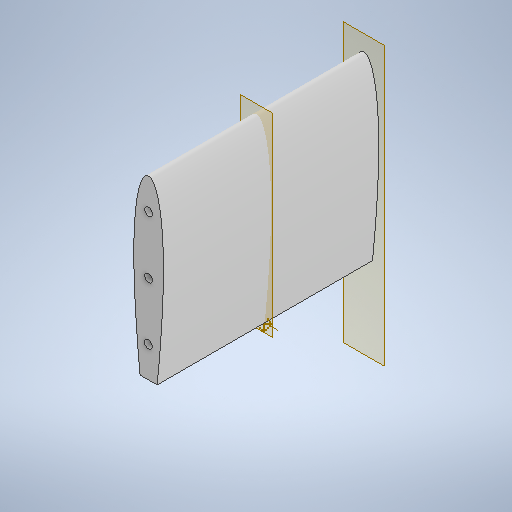
# Autodesk Inventor part: MiddleTailLeft
Saved by Autodesk Inventor 2025.2 (Build 292293000, 293)
## iProperties
Created: 2025-03-03
Part Number: MiddleTailLeft
Material: Generic
Document SubType Name: Modeling
Designer: georg
Density: 1 g/cm^3
Appearance: Default
Author: georg
Autodesk Inventor part; units mm, degrees
ref_plane "YZ Plane" through (0, 0, 0) normal (1, 0, 0) x (0, 1, 0)
ref_plane "XZ Plane" through (0, 0, 0) normal (0, 1, 0) x (-1, 0, 0)
ref_plane "XY Plane" through (0, 0, 0) normal (0, 0, 1) x (1, 0, 0)
ref_plane "Work Plane1" through (0, 0, 156.21) normal (0, 0, 1) x (1, 0, 0)
sketch "Sketch1" plane through (0, 0, 156.21) normal (0, 0, 1) x (1, 0, 0)
  line L0 (-0.0073, -145.66) -> (7.0407, -145.66)
  spline S0 degree 5 poles (7.0407, -145.66) (7.0573, -145.4958) (7.1327, -144.7531) (7.2665, -143.4248) (7.4579, -141.501) (7.705, -138.9697) (7.9903, -135.9869) (8.2715, -132.9695) (8.549, -129.922) (8.8215, -126.8457) (9.0881, -123.745) (9.3491, -120.6224) (9.6026, -117.4806) (9.8495, -114.3238) (10.0866, -111.1538) (10.3164, -107.9748) (10.5349, -104.7893) (10.7445, -101.6008) (10.942, -98.4123) (11.1277, -95.2267) (11.3009, -92.0477) (11.4615, -88.8777) (11.6069, -85.7208) (11.739, -82.5791) (11.8548, -79.4563) (11.9554, -76.3556) (12.039, -73.2792) (12.1057, -70.2316) (12.1549, -67.2141) (12.1854, -64.2311) (12.198, -61.2847) (12.1911, -58.378) (12.1652, -55.5142) (12.1197, -52.6956) (12.0539, -49.9253) (11.9681, -47.2063) (11.8622, -44.5404) (11.7355, -41.9312) (11.589, -39.3806) (11.4216, -36.8917) (11.2342, -34.4665) (11.0264, -32.1073) (10.7996, -29.817) (10.5524, -27.5973) (10.2861, -25.4503) (10.0015, -23.3788) (9.698, -21.3841) (9.3765, -19.469) (9.0379, -17.6343) (8.682, -15.8826) (8.3103, -14.2152) (7.9227, -12.634) (7.5202, -11.1404) (7.103, -9.7353) (6.6725, -8.4212) (6.2284, -7.198) (5.7722, -6.0677) (5.3036, -5.0307) (4.8237, -4.0882) (4.3332, -3.2402) (3.831, -2.4886) (3.3186, -1.832) (2.7948, -1.2726) (2.2592, -0.8103) (1.7116, -0.4465) (1.151, -0.1846) (0.5803, -0.0264) (0, 0.026) (-0.5803, -0.0264) (-1.151, -0.1846) (-1.7116, -0.4465) (-2.2592, -0.8103) (-2.7948, -1.2726) (-3.3186, -1.832) (-3.831, -2.4886) (-4.3332, -3.2402) (-4.8237, -4.0882) (-5.3036, -5.0307) (-5.7722, -6.0677) (-6.2284, -7.198) (-6.6725, -8.4212) (-7.103, -9.7353) (-7.5202, -11.1404) (-7.9227, -12.634) (-8.3103, -14.2152) (-8.682, -15.8826) (-9.0379, -17.6343) (-9.3765, -19.469) (-9.698, -21.3841) (-10.0015, -23.3788) (-10.2861, -25.4503) (-10.5524, -27.5973) (-10.7996, -29.817) (-11.0264, -32.1073) (-11.2342, -34.4665) (-11.4216, -36.8917) (-11.589, -39.3806) (-11.7355, -41.9312) (-11.8622, -44.5404) (-11.9681, -47.2063) (-12.0539, -49.9253) (-12.1197, -52.6956) (-12.1652, -55.5142) (-12.1911, -58.378) (-12.198, -61.2847) (-12.1854, -64.2311) (-12.1549, -67.2141) (-12.1057, -70.2316) (-12.039, -73.2792) (-11.9554, -76.3556) (-11.8548, -79.4563) (-11.739, -82.5791) (-11.6069, -85.7208) (-11.4615, -88.8777) (-11.3009, -92.0477) (-11.1277, -95.2267) (-10.942, -98.4123) (-10.7445, -101.6008) (-10.5349, -104.7893) (-10.3164, -107.9748) (-10.0866, -111.1538) (-9.8495, -114.3238) (-9.6026, -117.4806) (-9.3491, -120.6224) (-9.0881, -123.745) (-8.8215, -126.8457) (-8.549, -129.922) (-8.2715, -132.9695) (-7.9903, -135.9869) (-7.705, -138.9697) (-7.4579, -141.501) (-7.2665, -143.4248) (-7.1327, -144.7531) (-7.0573, -145.4958) (-7.0407, -145.66) knots 0.155732 0.155732 0.155732 0.155732 0.155732 0.155732 0.15748 0.163633 0.169829 0.176062 0.18233 0.188629 0.194957 0.201309 0.207683 0.214076 0.220484 0.226904 0.233333 0.239767 0.246204 0.25264 0.259072 0.265497 0.271912 0.278314 0.284699 0.291064 0.297407 0.303723 0.310011 0.316266 0.322485 0.328666 0.334804 0.340898 0.346943 0.352937 0.358876 0.364757 0.370576 0.376331 0.382017 0.387632 0.393172 0.398634 0.404014 0.409309 0.414515 0.419627 0.424644 0.42956 0.434371 0.439075 0.443667 0.448142 0.452498 0.456729 0.460831 0.464802 0.468638 0.472335 0.475892 0.479309 0.482586 0.485731 0.488751 0.491664 0.494492 0.497262 0.5 0.502738 0.505508 0.508336 0.511249 0.514269 0.517414 0.520691 0.524108 0.527665 0.531362 0.535198 0.539169 0.543271 0.547502 0.551858 0.556333 0.560925 0.565629 0.57044 0.575356 0.580373 0.585485 0.590691 0.595986 0.601366 0.606828 0.612368 0.617983 0.623669 0.629424 0.635243 0.641124 0.647063 0.653057 0.659102 0.665196 0.671334 0.677515 0.683734 0.689989 0.696277 0.702593 0.708936 0.715301 0.721686 0.728088 0.734503 0.740928 0.74736 0.753796 0.760233 0.766667 0.773096 0.779516 0.785924 0.792317 0.798691 0.805043 0.811371 0.81767 0.823938 0.830171 0.836367 0.84252 0.844268 0.844268 0.844268 0.844268 0.844268 0.844268
  line L1 (-7.0407, -145.66) -> (-0.0073, -145.66)
  point P0 (0, 0)
  point P1 (7.4123, -141.9502)
  point P2 (7.7005, -139.0014)
  point P3 (7.9858, -136.0158)
  point P4 (8.2674, -132.996)
  point P5 (8.545, -129.9456)
  point P6 (8.8177, -126.8669)
  point P7 (9.0847, -123.7634)
  point P8 (9.3456, -120.638)
  point P9 (9.5996, -117.4937)
  point P10 (9.8461, -114.3339)
  point P11 (10.084, -111.1614)
  point P12 (10.3132, -107.9795)
  point P13 (10.5325, -104.7913)
  point P14 (10.7416, -101.6)
  point P15 (10.9393, -98.4087)
  point P16 (11.125, -95.2205)
  point P17 (11.2983, -92.0386)
  point P18 (11.4584, -88.8661)
  point P19 (11.6043, -85.7063)
  point P20 (11.7358, -82.562)
  point P21 (11.8518, -79.4366)
  point P22 (11.952, -76.3331)
  point P23 (12.0355, -73.2544)
  point P24 (12.102, -70.204)
  point P25 (12.1508, -67.1842)
  point P26 (12.1812, -64.1986)
  point P27 (12.1932, -61.2498)
  point P28 (12.1861, -58.3408)
  point P29 (12.1597, -55.4746)
  point P30 (12.1136, -52.6538)
  point P31 (12.0473, -49.8813)
  point P32 (11.961, -47.1601)
  point P33 (11.8543, -44.4923)
  point P34 (11.7271, -41.8809)
  point P35 (11.5796, -39.3285)
  point P36 (11.4115, -36.8377)
  point P37 (11.2231, -34.4107)
  point P38 (11.0147, -32.0499)
  point P39 (10.7865, -29.758)
  point P40 (10.5384, -27.5369)
  point P41 (10.2709, -25.3886)
  point P42 (9.9848, -23.3158)
  point P43 (9.68, -21.3202)
  point P44 (9.3572, -19.404)
  point P45 (9.0168, -17.5687)
  point P46 (8.6594, -15.8163)
  point P47 (8.2857, -14.1486)
  point P48 (7.8961, -12.5673)
  point P49 (7.4914, -11.0738)
  point P50 (7.072, -9.6695)
  point P51 (6.6387, -8.3562)
  point P52 (6.1921, -7.1348)
  point P53 (5.7329, -6.0066)
  point P54 (5.2615, -4.9727)
  point P55 (4.7787, -4.0341)
  point P56 (4.2851, -3.1919)
  point P57 (3.7809, -2.4469)
  point P58 (3.267, -1.7995)
  point P59 (2.7438, -1.2509)
  point P60 (2.2116, -0.8012)
  point P61 (1.6709, -0.4509)
  point P62 (1.1219, -0.2006)
  point P63 (0.5647, -0.0502)
  point P64 (0, 0)
  point P65 (-0.5647, -0.0502)
  point P66 (-1.1219, -0.2006)
  point P67 (-1.6709, -0.4509)
  point P68 (-2.2116, -0.8012)
  point P69 (-2.7438, -1.2509)
  point P70 (-3.267, -1.7995)
  point P71 (-3.7809, -2.4469)
  point P72 (-4.2851, -3.1919)
  point P73 (-4.7787, -4.0341)
  point P74 (-5.2615, -4.9727)
  point P75 (-5.7329, -6.0066)
  point P76 (-6.1921, -7.1348)
  point P77 (-6.6387, -8.3562)
  point P78 (-7.072, -9.6695)
  point P79 (-7.4914, -11.0738)
  point P80 (-7.8961, -12.5673)
  point P81 (-8.2857, -14.1486)
  point P82 (-8.6594, -15.8163)
  point P83 (-9.0168, -17.5687)
  point P84 (-9.3572, -19.404)
  point P85 (-9.68, -21.3202)
  point P86 (-9.9848, -23.3158)
  point P87 (-10.2709, -25.3886)
  point P88 (-10.5384, -27.5369)
  point P89 (-10.7865, -29.758)
  point P90 (-11.0147, -32.0499)
  point P91 (-11.2231, -34.4107)
  point P92 (-11.4115, -36.8377)
  point P93 (-11.5796, -39.3285)
  point P94 (-11.7271, -41.8809)
  point P95 (-11.8543, -44.4923)
  point P96 (-11.961, -47.1601)
  point P97 (-12.0473, -49.8813)
  point P98 (-12.1136, -52.6538)
  point P99 (-12.1597, -55.4746)
  point P100 (-12.1861, -58.3408)
  point P101 (-12.1932, -61.2498)
  point P102 (-12.1812, -64.1986)
  point P103 (-12.1508, -67.1842)
  point P104 (-12.102, -70.204)
  point P105 (-12.0355, -73.2544)
  point P106 (-11.952, -76.3331)
  point P107 (-11.8518, -79.4366)
  point P108 (-11.7358, -82.562)
  point P109 (-11.6043, -85.7063)
  point P110 (-11.4584, -88.8661)
  point P111 (-11.2983, -92.0386)
  point P112 (-11.125, -95.2205)
  point P113 (-10.9393, -98.4087)
  point P114 (-10.7416, -101.6)
  point P115 (-10.5325, -104.7913)
  point P116 (-10.3132, -107.9795)
  point P117 (-10.084, -111.1614)
  point P118 (-9.8461, -114.3339)
  point P119 (-9.5996, -117.4937)
  point P120 (-9.3456, -120.638)
  point P121 (-9.0847, -123.7634)
  point P122 (-8.8177, -126.8669)
  point P123 (-8.545, -129.9456)
  point P124 (-8.2674, -132.996)
  point P125 (-7.9858, -136.0158)
  point P126 (-7.7005, -139.0014)
  point P127 (-7.4123, -141.9502)
  point P128 (-7.1218, -144.8592)
  dimension "d4" = 145.66
  constraints: 4 end point, 1 coincident, 1 horizontal, 132 other
  measures "d4" distance of point (0, 0) L0.start
extrude "Extrusion1" add sketch "Sketch1" along normal blind 177.62
sketch "Sketch2" plane through (0, 0, 156.21) normal (0, 0, 1) x (1, 0, 0)
  circle A0 centre (0, -25.4) radius 3.175
  circle A1 centre (-0.2097, -120.26) radius 3.175
  circle A2 centre (0, -72.8255) radius 3.175
  line L0 (-7.0407, -145.66) -> (7.0407, -145.66)
  point P0 (0, 0)
  dimension "d8" = 6.35
  dimension "d10" = 6.35
  dimension "d12" = 6.35
  dimension "d22" = 25.4
  dimension "d25" = 47.4345
  dimension "d28" = 25.4
  dimension "d29" = 47.4255
  constraints: 3 centre point, 2 end point, 1 other
  measures "d8" diameter of A0
  measures "d10" diameter of A1
  measures "d12" diameter of A2
  measures "d22" distance of point (0, 0) A0.centre
  measures "d25" vertical distance of A1.centre A2.centre
  measures "d28" distance from line of L0 A1.centre
  measures "d29" distance of A0.centre A2.centre
extrude "Extrusion2" cut sketch "Sketch2" along normal blind 25.4
ref_plane "Work Plane2" through (7.0407, -145.66, 245.02) normal (0, 0, 1) x (1, 0, 0)
mirror "Mirror1" about plane through (7.0407, -145.66, 245.02) normal (0, 0, 1) of "Extrusion2"
body "Solid1"
